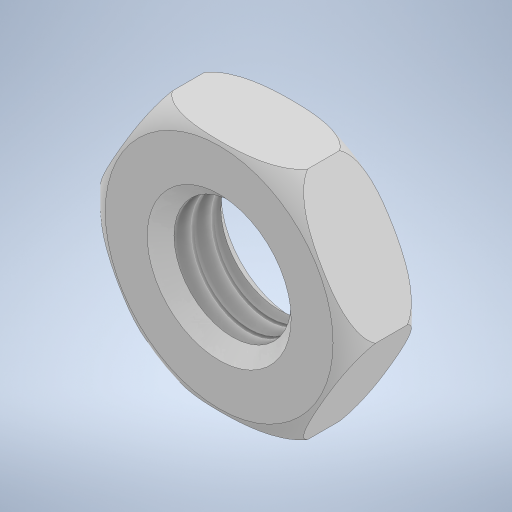
# Autodesk Inventor part: somun
Saved by Autodesk Inventor 2023.2 (Build 272271000, 271)
## iProperties
Created: 2022-11-27
Part Number: somun
Material: Generic
Document SubType Name: Modeling
Designer: omrfrkmll
Density: 1 g/cm^3
Appearance: Default
Author: omrfrkmll
Autodesk Inventor part; units mm, degrees
ref_plane "YZ Plane" through (0, 0, 0) normal (1, 0, 0) x (0, 1, 0)
ref_plane "XZ Plane" through (0, 0, 0) normal (0, 1, 0) x (-1, 0, 0)
ref_plane "XY Plane" through (0, 0, 0) normal (0, 0, 1) x (1, 0, 0)
sketch "Sketch1" plane through (0, 0, 0) normal (0, 0, 1) x (1, 0, 0)
  line L0 (-4.0776, 0) -> (11.9806, 0)
  line L1 (0, 5.675) -> (0, -5.0865)
  line L2 (-3.6188, 3.5) -> (4.159, 3.5)
  line L3 (-3.3522, -3.5) -> (4.4256, -3.5)
  line L4 (-1.2217, -4.8839) -> (-5.1106, 1.8518)
  line L5 (4.7072, -1.1531) -> (0.8183, 5.5827)
  line L6 (4.8405, 1.3839) -> (0.9516, -5.3518)
  line L7 (-1.355, 4.6531) -> (-5.2439, -2.0827)
  circle A0 centre (0, 0) radius 1.75
  point P0 (4.0415, 0)
  point P1 (2.0207, 3.5)
  point P2 (-2.0207, 3.5)
  point P3 (-4.0415, 0)
  point P4 (-2.0207, -3.5)
  point P5 (2.0207, -3.5)
  dimension "d0" = 7
  dimension "d3" = 360
  dimension "d5" = 3.5
  constraints: 16 end point, 4 horizontal, 2 vertical, 1 centre point, 1 coincident, 1 parallel, 20 other
  measures "d0" distance between parallel lines of L3 L2
  measures "d5" diameter of A0
extrude "Extrusion1" add sketch "Sketch1" along normal mid plane 2.2 contours L7 L2 L1 A0 L0 | L0 A0 L1 L3 L4 | L1 L2 L5 L0 A0 | A0 L0 L6 L3 L1
sketch "Sketch2" plane through (0, 0, 0) normal (0, 1, 0) x (-1, 0, 0)
  circle A0 centre (3.1105, -0.1599) radius 0.984
  line L0 (0, -2.0822) -> (0, 3.6497)
  line L1 (2.0207, -1.1) -> (4.0415, -1.1) projected
  line L2 (3.4011, -1.1) -> (4.0415, -1.1)
  line L3 (4.0415, -1.1) -> (4.0415, 0.1588)
  point P0 (0, 0)
  point P1 (4.0415, -0.4786)
  point P2 (2.8198, -1.1)
  dimension "d11" = 1.968
  dimension "d12" = 0.9401
  dimension "d13" = 0.931
  constraints: 6 end point, 2 point on circle, 1 centre point, 1 horizontal, 1 perpendicular, 1 point on line, 1 vertical
  measures "d11" diameter of A0
  measures "d12" distance from line of L1 A0.centre
  measures "d13" distance from line of L3 A0.centre
revolve "Revolution1" cut sketch "Sketch2" angle 360 about axis through (0, 0, -2.0822) along (0, 0, 1) picked at (3.9263, -0.8843) contours L3 L1 A0 | L1 A0
mirror "Mirror1" about plane through (0, 0, 0) normal (0, 0, 1) of "Revolution1"
thread "Thread1" size "M3.5x0.6" class "6H" standard "ANSI Metric M Profile" length 45
chamfer "Chamfer1" distance 0.4 angle 45 1 edges at (-1.75, 0, 1.1)
chamfer "Chamfer2" distance 0.4 angle 45 1 edges at (-1.75, 0, -1.1)
body "Solid1"
